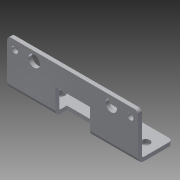
# Autodesk Inventor part: Mounting Bracket V1.500 - (toughbox-mini - sheet metal)
Saved by Autodesk Inventor 2013 (Build 170138000, 138)
## iProperties
Created: 2013-01-13
Part Number: Mounting Bracket V1.500 - (toughbox-mini - sheet metal)
Material: Aluminum 6061
Document SubType Name: Sheet Metal
Designer: Moses
Density: 2.71 g/cm^3
Flat Pattern Width: 6.19743 cm
Flat Pattern Length: 10.795 cm
Flat Pattern Area: 66.9013 cm^2
Sheet Metal Rule: Default
Sheet Metal Width: 2.440 in
Sheet Metal Length: 4.250 in
Sheet Metal Area: 10.370 in^2
Mass: 48.5197 g
Surface Area: 132.461 cm^2
Volume: 17.904 cm^3
Author: Moses
Autodesk Inventor part; units mm, degrees
ref_plane "YZ Plane" through (0, 0, 0) normal (1, 0, 0) x (0, 1, 0)
ref_plane "XZ Plane" through (0, 0, 0) normal (0, 1, 0) x (-1, 0, 0)
ref_plane "XY Plane" through (0, 0, 0) normal (0, 0, 1) x (1, 0, 0)
sketch "Sketch1" plane through (0, 0, 0) normal (0, 1, 0) x (-1, 0, 0)
  line L0 (0, 0) -> (107.95, 0)
  line L1 (107.95, 0) -> (107.95, 28.575)
  line L2 (107.95, 28.575) -> (0, 28.575)
  line L3 (0, 28.575) -> (0, 0)
  dimension "d0" = 107.95
  dimension "d1" = 28.575
  measures "d0" distance of L0.start L0.end
  measures "d1" distance of L0.end L1.end
extrude "Plate1" add sketch "Sketch1" along normal blind 3.175
sketch "Sketch2" plane through (0, 0, 25.4) normal (0, 0, 1) x (1, 0, 0)
  line L0 (-107.95, 0) -> (0, 0)
  line L1 (0, 0) -> (0, 38.1)
  line L2 (0, 38.1) -> (-107.95, 38.1)
  line L3 (-107.95, 38.1) -> (-107.95, 0)
  constraints: 6 end point, 1 horizontal, 1 perpendicular, 1 vertical
edge flange "Flange1" height 38.1 angle 90 thickness 3.175 bend radius 1.27 thickness toward (0, 0, 1) relief straight relief width 3.175 relief depth 1.5875 edges at (-53.975, 3.175, 28.575) wall of the first edge with corners at (-107.95, 0, 25.4) (0, 0, 25.4) (0, 38.1, 25.4) (-107.95, 38.1, 25.4)
bend "Bend1"
corner "Corner1"
sketch "Sketch3" plane through (-107.95, 38.1, 28.575) normal (0, 0, 1) x (1, 0, 0)
  line L0 (0, -33.655) -> (107.95, -33.655) projected
  line L1 (0, 0) -> (107.95, 0) projected
  line L2 (39.6875, -16.8275) -> (68.2625, -16.8275)
  line L3 (68.2625, -16.8275) -> (68.2625, -38.1)
  line L4 (68.2625, -38.1) -> (39.6875, -38.1)
  line L5 (39.6875, -38.1) -> (39.6875, -16.8275)
  line L6 (53.975, 0) -> (53.975, -33.655) construction
  line L7 (107.95, -38.1) -> (0, -38.1) construction
  point P0 (53.975, -16.8275)
  dimension "d18" = 28.575
  constraints: 10 end point, 4 midpoint, 2 parallel, 1 horizontal, 1 perpendicular, 1 point on line
  measures "d18" distance of L2.start L2.end
extrude "Cut1" cut sketch "Sketch3" against normal blind 9.525
sketch "Sketch4" plane through (0, 3.175, 0) normal (0, 1, 0) x (1, 0, 0)
  line L0 (-68.2625, -19.05) -> (-39.6875, -19.05) projected
  line L1 (0, 0) -> (0, -24.13) projected
  line L2 (-107.95, 0) -> (0, 0) projected
  line L3 (-107.95, -24.13) -> (-107.95, 0) projected
  line L4 (-107.95, -28.575) -> (0, -28.575) projected
  line L5 (-107.95, -12.7) -> (0, -12.7) construction
  circle A0 centre (-79.375, -12.7) radius 3.302
  circle A1 centre (-28.575, -12.7) radius 3.302
  line L6 (-53.975, -19.05) -> (-53.975, 0) construction
  dimension "d22" = 15.875
  dimension "d23" = 6.604
  dimension "d24" = 6.604
  dimension "d25" = 50.8
  dimension "d26" = 25.4
  constraints: 4 end point, 4 point on line, 2 centre point, 2 midpoint, 1 parallel
  measures "d22" distance between parallel lines of L4 L5
  measures "d23" diameter of A0
  measures "d24" diameter of A1
  measures "d25" distance of A1.centre A0.centre
  measures "d26" distance from line of A1.centre L6
extrude "Cut2" cut sketch "Sketch4" against normal blind 3.175
fillet "Corner Round1" radius 3.175 4 edges at (0, 38.1, 26.9875) (0, 1.5875, 0) (-107.95, 38.1, 26.9875) (-107.95, 1.5875, 0)
sketch "Sketch5" plane through (0, 4.445, 25.4) normal (0, 0, -1) x (-1, 0, 0)
  line L0 (5.856, 35.4838) -> (102.094, 35.4838) construction
  arc A0 (5.856, 35.4838) -> (-0.4733, 29.647) centre (5.856, 29.1338) ccw construction
  line L1 (-9.525, -81.9912) -> (-0.4733, 29.647) construction
  line L2 (-9.525, -83.6422) -> (-9.525, -81.9912) construction
  line L3 (-9.525, -83.6422) -> (117.475, -83.6422) construction
  line L4 (117.475, -81.9912) -> (117.475, -83.6422) construction
  line L5 (108.4233, 29.647) -> (117.475, -81.9912) construction
  arc A1 (108.4233, 29.647) -> (102.094, 35.4838) centre (102.094, 29.1338) ccw construction
  circle A2 centre (16.383, 26.4935) radius 2.0447 construction
  circle A3 centre (0, -62.4065) radius 2.5527 construction
  circle A4 centre (6.35, 26.4935) radius 2.5527 projected
  circle A5 centre (92.71, -62.4065) radius 2.5527 construction
  circle A6 centre (22.225, 26.4935) radius 2.5527 projected
  circle A7 centre (53.975, -44.0944) radius 14.2811 construction
  circle A8 centre (92.71, -15.9245) radius 5.5562 construction
  circle A9 centre (15.24, -41.3245) radius 5.5562 construction
  circle A10 centre (15.24, -15.9245) radius 5.5562 construction
  circle A11 centre (53.975, -3.3782) radius 11.1061 construction
  circle A12 centre (15.24, 9.4755) radius 5.5562 construction
  circle A13 centre (92.71, -41.3245) radius 5.5562 construction
  circle A14 centre (92.71, 9.4755) radius 5.5562 construction
  circle A15 centre (85.725, 26.4935) radius 2.5527 projected
  circle A16 centre (15.24, -62.4065) radius 2.5527 construction
  circle A17 centre (101.6, 26.4935) radius 2.5527 projected
  circle A18 centre (107.95, -62.4065) radius 2.5527 construction
  circle A19 centre (91.567, 26.4935) radius 2.0447 construction
  circle A20 centre (9.398, -62.4065) radius 2.0447 construction
  circle A21 centre (98.552, -62.4065) radius 2.0447 construction
  circle A22 centre (22.225, 26.4935) radius 4.7625
  circle A23 centre (85.725, 26.4935) radius 4.7625
  line L6 (0, 30.48) -> (0, 0) projected
  line L7 (107.95, 30.48) -> (107.95, 0) projected
  point P0 (0, -4.445)
  dimension "d34" = 9.525
  dimension "d35" = 9.525
  dimension "d36" = 22.225
  dimension "d37" = 22.225
  dimension "d38" = 6.35
  dimension "d39" = 6.35
  constraints: 2 centre point, 2 coincident
  measures "d34" diameter of A22
  measures "d35" diameter of A23
  measures "d36" distance from line of L7 A15.centre
  measures "d37" distance from line of L6 A6.centre
  measures "d38" distance from line of L6 A4.centre
  measures "d39" distance from line of L7 A17.centre
extrude "Cut3" cut sketch "Sketch5" against normal blind 3.175 contours A4 | A6 | A15 | A17 | A22 | A23
sketch "Sketch6" plane through (0, 3.175, 0) normal (0, 1, 0) x (1, 0, 0)
  circle A0 centre (-9.525, -12.7) radius 3.302 projected
  circle A1 centre (-98.425, -12.7) radius 3.302 projected
  point P0 (0, 0)
extrude "Cut4" cut sketch "Sketch6" against normal blind 3.175
ref_plane "Work Plane1" through (-53.975, 0, 24.13) normal (1, 0, 0) x (0, 0, -1)
equation "\"d24\" = d23"
equation "\"d26\" = 0.5 * d25"
equation "\"d27\" = Thickness"
equation "\"d35\" = d34"
equation "\"d30\" = Thickness"
equation "\"d32\" = Thickness"
equation "\"d4\" = BendReliefWidth"
equation "\"d5\" = BendReliefDepth"
equation "\"d6\" = MinimumRemnant"
equation "\"d7\" = BendRadius"
equation "\"d11\" = CornerReliefSize"
equation "\"d12\" = GapSize"
equation "\"d13\" = JacobiRadiusSize"
equation "\"BendRadius\" = Thickness"
equation "\"BendReliefWidth\" = Thickness"
equation "\"BendReliefDepth\" = 0.5 * Thickness"
equation "\"CornerReliefSize\" = 4 * Thickness"
equation "\"MinimumRemnant\" = 2 * Thickness"
equation "\"TransitionRadius\" = BendRadius"
equation "\"JacobiRadiusSize\" = BendRadius"
equation "\"GapSize\" = Thickness"
equation "\"d3\" = BendRadius"
equation "\"Thickness\" = 3.175"
body "Solid1"
